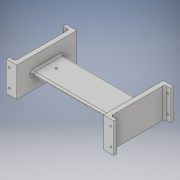
# Autodesk Inventor part: CenterThrusterBracket
Saved by Autodesk Inventor 2017 (Build 210142000, 142)
## iProperties
Created: 2017-08-29
Part Number: CenterThrusterBracket
Material: Generic
Document SubType Name: Modeling
Designer: tim38
Density: 1 g/cm^3
Appearance: Default
Author: tim38
Autodesk Inventor part; units mm, degrees
ref_plane "YZ Plane" through (0, 0, 0) normal (1, 0, 0) x (0, 1, 0)
ref_plane "XZ Plane" through (0, 0, 0) normal (0, 1, 0) x (-1, 0, 0)
ref_plane "XY Plane" through (0, 0, 0) normal (0, 0, 1) x (1, 0, 0)
sketch "Sketch1" plane through (0, 0, 0) normal (0, 1, 0) x (-1, 0, 0)
  line L0 (73.533, 25.4) -> (-73.533, 25.4)
  line L1 (-73.533, 25.4) -> (-73.533, -25.4)
  line L2 (-73.533, -25.4) -> (73.533, -25.4)
  line L3 (73.533, -25.4) -> (73.533, 25.4)
  line L4 (73.533, 25.4) -> (-73.533, -25.4) construction
  line L5 (-73.533, 25.4) -> (73.533, -25.4) construction
  circle A0 centre (57.15, 0) radius 1.7526
  circle A1 centre (-57.15, 0) radius 1.7526
  point P0 (0, 0)
  dimension "d0" = 147.066
  dimension "d1" = 50.8
  dimension "d2" = 57.15
  dimension "d3" = 3.5052
  dimension "d4" = 3.5052
  dimension "d5" = 57.15
  constraints: 12 end point, 2 centre point, 2 midpoint, 2 parallel, 1 horizontal, 1 perpendicular
  measures "d0" distance of L1.end L2.end
  measures "d1" distance of L0.end L1.end
  measures "d2" distance of A0.centre point (0, 0)
  measures "d3" diameter of A0
  measures "d4" diameter of A1
  measures "d5" distance of A1.centre point (0, 0)
extrude "Extrusion1" add sketch "Sketch1" along normal blind 6.35
fillet "Fillet2" radius 2.54 4 edges at (0, 0, 25.4) (0, 6.35, 25.4) (0, 0, -25.4) (0, 6.35, -25.4)
sketch "Sketch3" plane through (-73.533, 0, -22.86) normal (-1, 0, 0) x (0, 0, 1)
  line L0 (-27.94, 28.575) -> (73.66, 28.575)
  line L1 (73.66, 28.575) -> (73.66, -22.225)
  line L2 (73.66, -22.225) -> (-27.94, -22.225)
  line L3 (-27.94, -22.225) -> (-27.94, 28.575)
  line L4 (-27.94, 28.575) -> (73.66, -22.225) construction
  line L5 (73.66, 28.575) -> (-27.94, -22.225) construction
  point P0 (22.86, 0)
  point P1 (22.86, 3.175)
  dimension "d25" = 50.8
  dimension "d26" = 101.6
  dimension "d27" = 0
  dimension "d28" = 3.175
  constraints: 12 end point, 2 midpoint, 2 parallel, 1 horizontal, 1 perpendicular
  measures "d25" distance of L0.end L1.end
  measures "d26" distance of L1.end L2.end
  measures "d27" horizontal distance of point (22.86, 3.175) point (22.86, 0)
  measures "d28" distance of point (22.86, 0) point (22.86, 3.175)
extrude "Extrusion4" add sketch "Sketch3" along normal blind 7.62
sketch "Sketch4" plane through (-81.153, 0, -22.86) normal (-1, 0, 0) x (0, 0, 1)
  line L0 (73.66, 28.575) -> (73.66, -22.225) projected
  line L1 (73.66, 28.575) -> (68.58, 28.575)
  line L2 (68.58, 28.575) -> (68.58, -22.225)
  line L3 (68.58, -22.225) -> (73.66, -22.225)
  line L4 (73.66, -22.225) -> (73.66, 28.575)
  line L5 (-27.94, -22.225) -> (-27.94, 28.575) projected
  line L6 (73.66, 28.575) -> (-27.94, 28.575) projected
  line L7 (-27.94, -22.225) -> (-22.86, -22.225)
  line L8 (-22.86, -22.225) -> (-22.86, 28.575)
  line L9 (-22.86, 28.575) -> (-27.94, 28.575)
  line L10 (-27.94, 28.575) -> (-27.94, -22.225)
  point P0 (22.86, 0)
  dimension "d32" = 5.08
  dimension "d33" = 5.08
  constraints: 16 end point, 4 parallel, 2 horizontal, 2 perpendicular, 1 point on line
  measures "d32" distance of L0.start L1.end
  measures "d33" distance of L8.end L5.end
extrude "Extrusion5" add sketch "Sketch4" along normal blind 10.16
sketch "Sketch6" plane through (-73.533, -22.225, 50.8) normal (0, 0, 1) x (1, 0, 0)
  line L0 (-17.78, 0) -> (-17.78, 50.8) projected
  line L1 (0, 50.8) -> (-17.78, 50.8) projected
  line L2 (0, 0) -> (-17.78, 0) projected
  point P0 (73.533, 22.225)
  point P1 (-12.7, 40.64)
  point P2 (-12.7, 10.16)
  dimension "d36" = 5.08
  dimension "d37" = 10.16
  dimension "d38" = 10.16
  dimension "d39" = 5.08
  measures "d36" distance from line of L0 point (-12.7, 40.64)
  measures "d37" distance from line of L1 point (-12.7, 40.64)
  measures "d38" distance from line of L2 point (-12.7, 10.16)
  measures "d39" distance from line of L0 point (-12.7, 10.16)
hole "Hole1" at (-86.233, 18.415, 50.8) at (-86.233, -12.065, 50.8) direction (0, 0, -1) diameter 3.15 end through all
fillet "Fillet3" radius 3.175 2 edges at (-81.153, 3.175, -45.72) (-81.153, 3.175, 45.72)
ref_plane "Work Plane2" through (0, 0, 22.86) normal (1, 0, 0) x (0, 0, -1)
mirror "Mirror2" about plane through (0, 0, 22.86) normal (1, 0, 0) of "Extrusion4", "Hole1", "Fillet3", "Extrusion5"
fillet "Fillet4" radius 3.175 16 edges at (73.533, 5.6061, -24.6561) (73.533, 3.175, -25.4) (73.533, 0.7439, -24.6561) (73.533, 0, 0) (73.533, 0.7439, 24.6561) (73.533, 3.175, 25.4) (73.533, 5.6061, 24.6561) (73.533, 6.35, 0) (-73.533, 5.6061, 24.6561) (-73.533, 3.175, 25.4) (-73.533, 0.7439, 24.6561) (-73.533, 0, 0) (-73.533, 0.7439, -24.6561) (-73.533, 3.175, -25.4) (-73.533, 5.6061, -24.6561) (-73.533, 6.35, 0)
equation "\"d5\" = d2"
equation "\"d33\" = d32"
equation "\"d38\" = d37"
equation "\"d39\" = d36"
body "Solid1"
